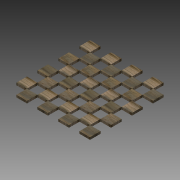
# Autodesk Inventor part: Board Piece 1
Saved by Autodesk Inventor 2015 SP1 (Build 190203100, 203)
## iProperties
Created: 2015-06-11
Part Number: Board Piece 1
Material: Generic
Document SubType Name: Modeling
Designer: Nathan
Density: 1 g/cm^3
Appearance: Driftwood
Author: Nathan
Autodesk Inventor part; units mm, degrees
ref_plane "YZ Plane" through (0, 0, 0) normal (1, 0, 0) x (0, 1, 0)
ref_plane "XZ Plane" through (0, 0, 0) normal (0, 1, 0) x (-1, 0, 0)
ref_plane "XY Plane" through (0, 0, 0) normal (0, 0, 1) x (1, 0, 0)
sketch "Sketch1" plane through (0, 0, 0) normal (0, 1, 0) x (-1, 0, 0)
  line L0 (180, 180) -> (-180, 180)
  line L1 (-180, 180) -> (-180, -180)
  line L2 (-180, -180) -> (180, -180)
  line L3 (180, -180) -> (180, 180)
  line L4 (180, 180) -> (-180, -180) construction
  line L5 (-180, 180) -> (180, -180) construction
  point P0 (0, 0)
  dimension "d0" = 360
  dimension "d1" = 360
  constraints: 12 end point, 2 midpoint, 2 parallel, 1 horizontal, 1 perpendicular
  measures "d0" distance of L2.end L1.end
  measures "d1" distance of L1.end L0.end
extrude "Extrusion1" add sketch "Sketch1" along normal blind 10
sketch "Sketch2" plane through (0, 10, 0) normal (0, 1, 0) x (1, 0, 0)
  line L0 (-180, -180) -> (-135, -180)
  line L1 (-135, -180) -> (-135, -135)
  line L2 (-135, -135) -> (-180, -135)
  line L3 (-180, -135) -> (-180, -180)
  line L4 (-180, -90) -> (-135, -90)
  line L5 (-135, -90) -> (-135, -45)
  line L6 (-135, -45) -> (-180, -45)
  line L7 (-180, -45) -> (-180, -90)
  line L8 (-180, 0) -> (-135, 0)
  line L9 (-135, 0) -> (-135, 45)
  line L10 (-135, 45) -> (-180, 45)
  line L11 (-180, 45) -> (-180, 0)
  line L12 (-180, 90) -> (-135, 90)
  line L13 (-135, 90) -> (-135, 135)
  line L14 (-135, 135) -> (-180, 135)
  line L15 (-180, 135) -> (-180, 90)
  line L16 (-90, -180) -> (-45, -180)
  line L17 (-45, -180) -> (-45, -135)
  line L18 (-45, -135) -> (-90, -135)
  line L19 (-90, -135) -> (-90, -180)
  line L20 (-90, -90) -> (-45, -90)
  line L21 (-45, -90) -> (-45, -45)
  line L22 (-45, -45) -> (-90, -45)
  line L23 (-90, -45) -> (-90, -90)
  line L24 (-90, 0) -> (-45, 0)
  line L25 (-45, 0) -> (-45, 45)
  line L26 (-45, 45) -> (-90, 45)
  line L27 (-90, 45) -> (-90, 0)
  line L28 (-90, 90) -> (-45, 90)
  line L29 (-45, 90) -> (-45, 135)
  line L30 (-45, 135) -> (-90, 135)
  line L31 (-90, 135) -> (-90, 90)
  line L32 (0, -180) -> (45, -180)
  line L33 (45, -180) -> (45, -135)
  line L34 (45, -135) -> (0, -135)
  line L35 (0, -135) -> (0, -180)
  line L36 (0, -90) -> (45, -90)
  line L37 (45, -90) -> (45, -45)
  line L38 (45, -45) -> (0, -45)
  line L39 (0, -45) -> (0, -90)
  line L40 (0, 0) -> (45, 0)
  line L41 (45, 0) -> (45, 45)
  line L42 (45, 45) -> (0, 45)
  line L43 (0, 45) -> (0, 0)
  line L44 (0, 90) -> (45, 90)
  line L45 (45, 90) -> (45, 135)
  line L46 (45, 135) -> (0, 135)
  line L47 (0, 135) -> (0, 90)
  line L48 (90, -180) -> (135, -180)
  line L49 (135, -180) -> (135, -135)
  line L50 (135, -135) -> (90, -135)
  line L51 (90, -135) -> (90, -180)
  line L52 (90, -90) -> (135, -90)
  line L53 (135, -90) -> (135, -45)
  line L54 (135, -45) -> (90, -45)
  line L55 (90, -45) -> (90, -90)
  line L56 (90, 0) -> (135, 0)
  line L57 (135, 0) -> (135, 45)
  line L58 (135, 45) -> (90, 45)
  line L59 (90, 45) -> (90, 0)
  line L60 (90, 90) -> (135, 90)
  line L61 (135, 90) -> (135, 135)
  line L62 (135, 135) -> (90, 135)
  line L63 (90, 135) -> (90, 90)
  line L64 (-135, -135) -> (-90, -135)
  line L65 (-90, -135) -> (-90, -90)
  line L66 (-90, -90) -> (-135, -90)
  line L67 (-135, -90) -> (-135, -135)
  line L68 (-135, -45) -> (-90, -45)
  line L69 (-90, -45) -> (-90, 0)
  line L70 (-90, 0) -> (-135, 0)
  line L71 (-135, 0) -> (-135, -45)
  line L72 (-135, 45) -> (-90, 45)
  line L73 (-90, 45) -> (-90, 90)
  line L74 (-90, 90) -> (-135, 90)
  line L75 (-135, 90) -> (-135, 45)
  line L76 (-135, 135) -> (-90, 135)
  line L77 (-90, 135) -> (-90, 180)
  line L78 (-90, 180) -> (-135, 180)
  line L79 (-135, 180) -> (-135, 135)
  line L80 (-45, -135) -> (0, -135)
  line L81 (0, -135) -> (0, -90)
  line L82 (0, -90) -> (-45, -90)
  line L83 (-45, -90) -> (-45, -135)
  line L84 (-45, -45) -> (0, -45)
  line L85 (0, -45) -> (0, 0)
  line L86 (0, 0) -> (-45, 0)
  line L87 (-45, 0) -> (-45, -45)
  line L88 (-45, 45) -> (0, 45)
  line L89 (0, 45) -> (0, 90)
  line L90 (0, 90) -> (-45, 90)
  line L91 (-45, 90) -> (-45, 45)
  line L92 (-45, 135) -> (0, 135)
  line L93 (0, 135) -> (0, 180)
  line L94 (0, 180) -> (-45, 180)
  line L95 (-45, 180) -> (-45, 135)
  line L96 (45, -135) -> (90, -135)
  line L97 (90, -135) -> (90, -90)
  line L98 (90, -90) -> (45, -90)
  line L99 (45, -90) -> (45, -135)
  line L100 (45, -45) -> (90, -45)
  line L101 (90, -45) -> (90, 0)
  line L102 (90, 0) -> (45, 0)
  line L103 (45, 0) -> (45, -45)
  line L104 (45, 45) -> (90, 45)
  line L105 (90, 45) -> (90, 90)
  line L106 (90, 90) -> (45, 90)
  line L107 (45, 90) -> (45, 45)
  line L108 (45, 135) -> (90, 135)
  line L109 (90, 135) -> (90, 180)
  line L110 (90, 180) -> (45, 180)
  line L111 (45, 180) -> (45, 135)
  line L112 (135, -135) -> (180, -135)
  line L113 (180, -135) -> (180, -90)
  line L114 (180, -90) -> (135, -90)
  line L115 (135, -90) -> (135, -135)
  line L116 (135, -45) -> (180, -45)
  line L117 (180, -45) -> (180, 0)
  line L118 (180, 0) -> (135, 0)
  line L119 (135, 0) -> (135, -45)
  line L120 (135, 45) -> (180, 45)
  line L121 (180, 45) -> (180, 90)
  line L122 (180, 90) -> (135, 90)
  line L123 (135, 90) -> (135, 45)
  line L124 (135, 135) -> (180, 135)
  line L125 (180, 135) -> (180, 180)
  line L126 (180, 180) -> (135, 180)
  line L127 (135, 180) -> (135, 135)
  dimension "d4" = 45
  dimension "d5" = 45
  dimension "d8" = 90
  dimension "d11" = 90
  dimension "d18" = 45
  dimension "d19" = 45
  dimension "d20" = 90
  dimension "d21" = 90
  constraints: 256 end point, 4 collinear, 4 horizontal, 4 parallel, 2 perpendicular, 2 vertical, 236 other
  measures "d4" distance of L2.end L1.end
  measures "d5" distance of L1.end L0.end
  measures "d8" distance of L1.end L5.end
  measures "d11" distance of L1.end L17.end
  measures "d18" distance of L66.end L65.end
  measures "d19" distance of L65.end L64.end
  measures "d20" distance of L65.end L69.end
  measures "d21" distance of L65.end L81.end
extrude "Extrusion2" cut sketch "Sketch2" against normal blind 10 contours L3 L2 L1 L0 | L127 L126 L125 L124 | L67 L66 L65 L64 | L18 L17 L16 L19 | L4 L7 L6 L5 | L83 L82 L81 L80 | L23 L22 L21 L20 | L71 L70 L69 L68 | L34 L33 L32 L35 | L8 L11 L10 L9 | L99 L98 L97 L96 | L39 L38 L37 L36 | L87 L86 L85 L84 | L27 L26 L25 L24 | L75 L74 L73 L72 | L50 L49 L48 L51 | L12 L15 L14 L13 | L115 L114 L113 L112 | L55 L54 L53 L52 | L103 L102 L101 L100 | L43 L42 L41 L40 | L91 L90 L89 L88 | L31 L30 L29 L28 | L79 L78 L77 L76 | L119 L118 L117 L116 | L59 L58 L57 L56 | L107 L106 L105 L104 | L47 L46 L45 L44 | L95 L94 L93 L92 | L123 L122 L121 L120 | L63 L62 L61 L60 | L111 L110 L109 L108
body "Solid1"
